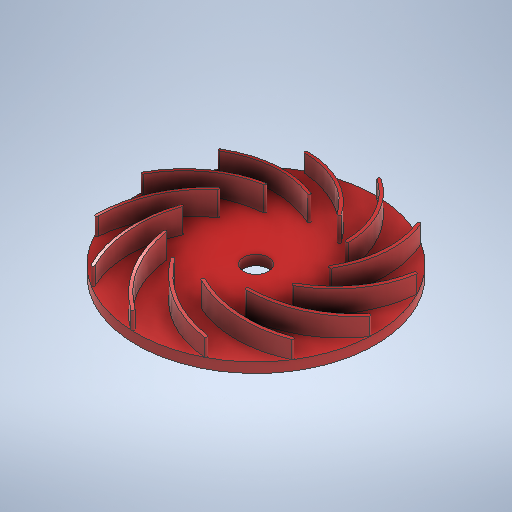
# Autodesk Inventor part: Rodete_4000RPM_2LS
Saved by Autodesk Inventor 2025.3 (Build 293356000, 356)
## iProperties
Created: 2025-11-12
Part Number: Rodete_4000RPM_2LS
Material: Generic
Document SubType Name: Modeling
Designer: juanm
Density: 1 g/cm^3
Appearance: Default
Author: juanm
Autodesk Inventor part; units mm, degrees
ref_plane "YZ Plane" through (0, 0, 0) normal (1, 0, 0) x (0, 1, 0)
ref_plane "XZ Plane" through (0, 0, 0) normal (0, 1, 0) x (-1, 0, 0)
ref_plane "XY Plane" through (0, 0, 0) normal (0, 0, 1) x (1, 0, 0)
sketch "Sketch1" plane through (0, 0, 0) normal (0, 1, 0) x (-1, 0, 0)
  circle A0 centre (0, 0) radius 24
  dimension "d0" = 48
  constraints: 1 centre point, 1 coincident
  measures "d0" diameter of A0
extrude "Extrusion1" add sketch "Sketch1" along normal blind 2
sketch "Sketch2" plane through (0, 2, 0) normal (0, 1, 0) x (1, 0, 0)
  circle A0 centre (0, 0) radius 24 projected
  circle A1 centre (0, 0) radius 13 construction
  line L0 (0, 0) -> (-24, 0)
  circle A2 centre (0, 0) radius 24 projected
  line L1 (0, 0) -> (-4.9958, 12.0017) construction
  line L2 (-4.9958, 12.0017) -> (-24, 0) construction
  line L3 (-8.6898, 9.6689) -> (0, 0) construction
  line L4 (-8.6898, 9.6689) -> (-6.3115, -11.053) construction
  line L5 (-24, 0) -> (-6.3115, -11.053) construction
  arc A3 (-8.2641, 9.7133) -> (-24, 0) centre (-6.3115, -11.053) ccw
  arc A4 (-8.3203, 10.3107) -> (-23.9732, 1.1332) centre (-6.3115, -11.053) ccw
  circle A5 centre (-23.6775, 1.0334) radius 0.3
  circle A6 centre (-8.2922, 10.012) radius 0.3
  point P0 (-23.4312, 0.862)
  point P1 (-23.9237, 1.2047)
  dimension "d3" = 26
  dimension "d4" = 67.4
  dimension "d6" = 35.4
  dimension "d7" = 32
  dimension "d8" = 0.6
  constraints: 12 end point, 11 point on circle, 5 centre point, 5 tangent, 4 point on line, 3 coincident, 1 horizontal
  measures "d3" diameter of A1
  measures "d4" angle of L0 L1
  measures "d6" angle of L4 L3
  measures "d7" angle of L5 L0
  measures "d8" radial gap between concentric circles of A3 A4
extrude "Extrusion2" add sketch "Sketch2" along normal blind 6.5 contours A5 | A4 A6 A3 A5 | A6
pattern_circular "Circular Pattern1" count 12 over 360 about axis through (0, -10, 0) along (0, 1, 0) of "Extrusion2"
sketch "Sketch3" plane through (0, 2, 0) normal (0, 1, 0) x (1, 0, 0)
  circle A0 centre (0, 0) radius 2.5
  dimension "d14" = 5
  constraints: 1 centre point, 1 coincident
  measures "d14" diameter of A0
extrude "Extrusion3" cut sketch "Sketch3" against normal through all
sketch "Sketch4" plane through (0, 0, 0) normal (0, 0, 1) x (1, 0, 0)
  line L0 (0, 0) -> (0, 8.5)
  line L1 (24, 0) -> (-24, 0) projected
  line L2 (0, 0) -> (-24, 0)
  line L3 (-24, 0) -> (-24, 2)
  line L4 (-24, 2) -> (-24, 5.5)
  line L5 (0.862, 2) -> (0.862, 8.5) projected
  line L6 (0, 8.5) -> (-24, 5.5)
  line L7 (-24, 5.5) -> (-24, 8.5)
  line L8 (-24, 8.5) -> (0, 8.5)
  dimension "d17" = 8.5
  dimension "d18" = 2
  dimension "d19" = 3.5
  constraints: 14 end point, 2 vertical, 1 collinear, 1 horizontal, 1 perpendicular, 1 point on line
  measures "d17" distance of L0.start L0.end
  measures "d18" distance of L1.end L3.end
  measures "d19" distance of L3.end L4.end
revolve "Revolution1" cut sketch "Sketch4" angle 360 about axis through (0, 0, 0) along (0, 1, 0) contours L6 L7 L8
body "Solid1"
